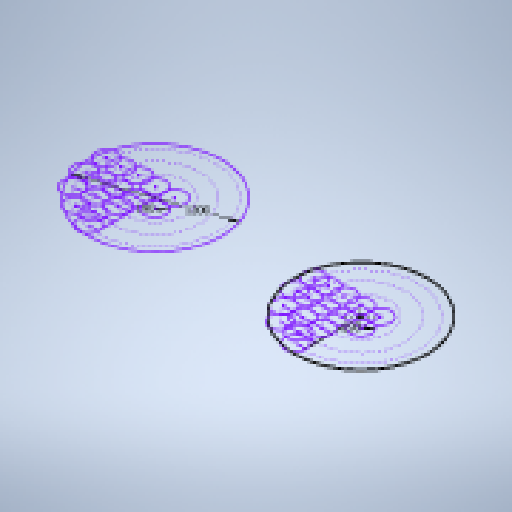
# Autodesk Inventor part: PNS 751 DIM filter-distribution-system 1200
Saved by Autodesk Inventor 2025.1 (Build 291241020, 241B)
## iProperties
Created: 2025-06-24
Part Number: PNS 751 DIM filter-distribution-system 1200
Material: Generic
Document SubType Name: Modeling
Designer: user
Density: 1 g/cm^3
Appearance: Default
Sheet Metal Rule: Default
Author: user
Autodesk Inventor part; units mm, degrees
ref_plane "YZ Plane" through (0, 0, 0) normal (1, 0, 0) x (0, 1, 0)
ref_plane "XZ Plane" through (0, 0, 0) normal (0, 1, 0) x (-1, 0, 0)
ref_plane "XY Plane" through (0, 0, 0) normal (0, 0, 1) x (1, 0, 0)
sketch "Sketch1" plane through (0, 0, 0) normal (0, 0, 1) x (1, 0, 0)
  circle A0 centre (0, 0) radius 600
  circle A1 centre (0, 0) radius 594
  dimension "d0" = 1200
  dimension "d1" = 6
  constraints: 2 centre point, 1 coincident
  measures "d0" diameter of A0
  measures "d1" radial gap between concentric circles of A0 A1
extrude "Extrusion1" add sketch "Sketch1" along normal blind 10
sketch "Sketch2" plane through (0, 0, 0) normal (0, 0, 1) x (1, 0, 0)
  circle A0 centre (0, 0) radius 519.1606 construction
  circle A1 centre (0, 0) radius 400.2566 construction
  circle A2 centre (0, 0) radius 253.9947 construction
  circle A3 centre (88.092, -88.092) radius 95
  circle A4 centre (-88.092, -88.092) radius 95
  circle A5 centre (-88.092, 88.092) radius 95
  circle A6 centre (88.092, 88.092) radius 95
  line L0 (88.092, 88.092) -> (-88.092, 88.092)
  line L1 (-88.092, 88.092) -> (-88.092, -88.092)
  line L2 (-88.092, -88.092) -> (88.092, -88.092)
  line L3 (88.092, -88.092) -> (88.092, 88.092)
  line L4 (88.092, 88.092) -> (-88.092, -88.092) construction
  line L5 (-88.092, 88.092) -> (88.092, -88.092) construction
  circle A7 centre (-238.2291, -88.092) radius 95
  circle A8 centre (-390.4422, -88.092) radius 95
  circle A9 centre (-511.6322, -88.092) radius 95
  circle A10 centre (-87.705, -267.7445) radius 95
  circle A11 centre (-162.3325, -405.1177) radius 95
  circle A12 centre (-88.092, -504.0772) radius 95
  circle A13 centre (-260.3738, -267.7445) radius 95
  circle A14 centre (-431.4198, -267.7445) radius 95
  circle A15 centre (-324.6649, -405.1177) radius 95
  circle A16 centre (-238.2291, 88.092) radius 95
  circle A17 centre (-390.4422, 88.092) radius 95
  circle A18 centre (-511.6322, 88.092) radius 95
  circle A19 centre (-1861.1768, 0.0383) radius 542.9574 construction
  circle A20 centre (-1861.1768, 0.0383) radius 405.4794 construction
  circle A21 centre (-1861.1768, 0.0383) radius 269.7641 construction
  circle A22 centre (-1775.4927, -88.092) radius 95
  circle A23 centre (-1951.6767, -81.9043) radius 95
  circle A24 centre (-1951.6767, 88.092) radius 95
  circle A25 centre (-1775.4927, 88.092) radius 95
  circle A26 centre (-2114.3969, -92.9793) radius 95
  circle A27 centre (-2253.4911, -102.4463) radius 95
  circle A28 centre (-2392.469, -111.9053) radius 95
  circle A29 centre (-1965.2761, -233.3106) radius 95
  circle A30 centre (-2023.09, -395.2734) radius 95
  circle A31 centre (-1952.9721, -514.2874) radius 95
  circle A32 centre (-2142.1114, -260.3738) radius 95
  circle A33 centre (-2321.5381, -287.8336) radius 95
  circle A34 centre (-2160.7174, -418.8379) radius 95
  circle A35 centre (-2111.9164, 99.5488) radius 95
  circle A36 centre (-2257.0071, 87.9697) radius 95
  circle A37 centre (-2396.4416, 91.1115) radius 95
  line L6 (-1861.1768, 0.0383) -> (-1861.1768, -542.9191)
  line L7 (-1861.1768, -75.7448) -> (-2392.469, -111.9053)
  line L8 (-1861.1768, -217.379) -> (-2321.5381, -287.8336)
  circle A38 centre (-1861.1768, 0.0383) radius 600
  line L9 (-1861.1768, -367.5508) -> (-2160.7174, -418.8379)
  line L10 (-1952.9721, -514.2874) -> (-1861.1768, -514.2874)
  line L11 (-88.092, -88.092) -> (-511.6322, -88.092)
  line L12 (0, 0) -> (0, -504.0772)
  line L13 (0, -504.0772) -> (-88.092, -504.0772)
  line L14 (0, -405.1177) -> (-324.6649, -405.1177)
  line L15 (0, -267.7445) -> (-431.4198, -267.7445)
  dimension "d4" = 190
  dimension "d5" = 190
  dimension "d6" = 1200
  constraints: 39 centre point, 32 end point, 30 equal radius, 20 point on line, 15 point on circle, 12 coincident, 6 perpendicular, 4 midpoint, 2 horizontal, 2 parallel, 1 vertical
  measures "d4" diameter of A3
  measures "d5" diameter of A22
  measures "d6" diameter of A38
equation "\"BendRadius\" = Thickness"
equation "\"BendReliefWidth\" = Thickness"
equation "\"BendReliefDepth\" = 0.5 * Thickness"
equation "\"CornerReliefSize\" = 4 * Thickness"
equation "\"MinimumRemnant\" = 2 * Thickness"
equation "\"TransitionRadius\" = BendRadius"
equation "\"JacobiRadiusSize\" = BendRadius"
equation "\"GapSize\" = Thickness"
equation "\"Thickness\" = 3.048"
body "Solid1"
